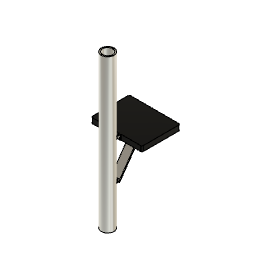
Seat_rod v5 (Autodesk Fusion 360 design; units mm, degrees)
Autodesk Fusion 360 part; units mm, degrees
sketch "草图1" plane through (0, 0, 0) normal (0, 0, 1) x (1, 0, 0)
  circle A0 centre (0, 0) radius 25
  dimension "d1" = 50
  constraint coincident A0.centre origin
  measures "d1" diameter of A0
extrude "拉伸1" add sketch "草图1" along normal mid plane 600 makes body 1
sketch "草图2" plane through (0, 0, 0) normal (0, 0, 1) x (1, 0, 0)
  line L0 (-10, 23) -> (-10, 35)
  line L1 (-10, 35) -> (10, 35)
  line L2 (10, 35) -> (10, 23)
  circle A0 centre (0, 0) radius 25
  circle A1 centre (0, 0) radius 25.0799
  dimension "d4" = 12
  dimension "d5" = 20
  dimension "d6" = 35
  dimension "d7" = 23
  dimension "d8" = 10
  constraint vertical L0
  constraint perpendicular L0 L1
  constraint perpendicular L1 L2
  constraint concentric A0 A1
  constraint coincident L2.end A1
  measures "d4" distance of L1.end L2.end
  measures "d5" distance of L0.end L1.end
  measures "d6" distance of A0.centre L1
  measures "d7" vertical distance of A0.centre L0.start
  measures "d8" horizontal distance of A0.centre L0.start
extrude "拉伸2" add sketch "草图2" along normal mid plane 12 separate body contours L0 L1 L2 A1 makes body 2
sketch "草图3" plane through (-10, 0, 0) normal (-1, 0, 0) x (0, -1, 0)
  line L0 (-23, -6) -> (-23, 6)
  line L1 (-23, 6) -> (-35, 6)
  line L2 (-35, 6) -> (-35, -6)
  line L3 (-35, -6) -> (-23, -6)
  circle A0 centre (-30, 0) radius 3
  line L4 (-1.75, 0) -> (-22.5, 0)
  dimension "d11" = 6
  dimension "d12" = 30
  constraint coincident A0.centre L4
  measures "d11" diameter of A0
  measures "d12" distance of origin A0.centre
extrude "拉伸3" cut sketch "草图3" against normal blind 20 contours A0 bodies 2
fillet "圆角1" radius 6 2 edges at (0, 35, 6) (0, 35, -6) on bodies 2
sketch "草图1 (2)" plane through (0, 0, 0) normal (1, 0, 0) x (0, 1, 0) in component "椅子"
  circle A0 centre (30, 0) radius 3
extrude "拉伸1'" add sketch "草图1 (2)" along normal mid plane 36 separate body makes body 3 in component "椅子"
sketch "草图1 (3)" plane through (0, 0, 0) normal (1, 0, 0) x (0, 1, 0) in component "支撑"
ref_plane "工作平面1" through (0, 0, -150) normal (0, 0, 1) x (1, 0, 0)
sketch "草图4" plane through (0, 0, -150) normal (0, 0, 1) x (1, 0, 0)
  circle A0 centre (0, 0) radius 25
  line L0 (-10, 29) -> (10, 29)
  line L1 (10, 29) -> (10, 23)
  arc A1 (10, 23) -> (-10, 23) centre (0, 0) ccw
  line L2 (-10, 23) -> (-10, 29)
  line L3 (-10, 29) -> (-10, 35)
  line L4 (-10, 29) -> (10, 29)
  line L5 (10, 35) -> (10, 29)
  line L6 (10, 29) -> (-10, 29)
  line L7 (10, 35) -> (-10, 35)
  constraint coincident L5.start L7.start
  constraint coincident L3.end L7.end
extrude "拉伸4" add sketch "草图4" along normal mid plane 10 separate body contours L0 L3 L4 L5 L6 L7 | L0 L1 A1 L2 L4 L6 makes body 4
sketch "草图8" plane through (0, 0, 0) normal (0, 0, 1) x (1, 0, 0) in component "椅子"
  line L0 (-10, 29) -> (-10, 35)
  line L1 (-10, 29) -> (10, 29)
  line L2 (10, 35) -> (10, 29)
  line L3 (10, 29) -> (-10, 29)
  line L4 (18, 33) -> (18, 35)
  line L5 (18, 35) -> (100, 35)
  line L6 (100, 35) -> (100, 185)
  line L7 (100, 185) -> (-100, 185)
  line L8 (-100, 185) -> (-100, 35)
  line L9 (-100, 35) -> (-18, 35)
  line L10 (-18, 35) -> (-18, 33)
  line L11 (-18, 33) -> (-10, 33)
  line L12 (-10, 35) -> (10, 35)
  line L13 (10, 33) -> (18, 33)
  line L14 (0, 1.75) -> (0, 22.5)
  dimension "d65" = 200
  dimension "d67" = 2
  dimension "d68" = 2
  dimension "d69" = 82
  dimension "d70" = 82
  dimension "d71" = 35
  dimension "d72" = 185
  dimension "d73" = 35
  constraint perpendicular L3 L4
  constraint perpendicular L4 L5
  constraint perpendicular L3 L6
  constraint perpendicular L8 L9
  constraint perpendicular L9 L10
  constraint coincident L0 L11.end
  constraint perpendicular L0 L11
  constraint coincident L0.end L12.start
  constraint coincident L2.start L12.end
  constraint coincident L2 L13.start
  constraint perpendicular L4 L13
  constraint symmetric L6 L8 L14
  constraint parallel L7 L9
  measures "d65" distance of L6.end L7.end
  measures "d67" distance of L9.end L10.end
  measures "d68" distance of L4.start L4.end
  measures "d69" distance of L4.end L5.end
  measures "d70" distance of L8.end L9.end
  measures "d71" distance of origin L9
  measures "d72" distance of origin L7
  measures "d73" distance of L5 origin
extrude "拉伸5" add sketch "草图8" along normal mid plane 20 separate body contours L0 L2 L4 L5 L6 L7 L8 L9 L10 L11 L12 L13 makes body 5 in component "椅子"
fillet "圆角4" radius 5 4 edges at (-100, 35, 0) (-100, 185, 0) (100, 185, 0) (100, 35, 0) on bodies 5 in component "椅子"
fillet "圆角2" radius 5 2 edges at (0, 35, -145) (0, 35, -155) on bodies 4
sketch "草图5" plane through (-10, 0, 0) normal (-1, 0, 0) x (0, -1, 0)
  arc A0 (-30, -145) -> (-30, -155) centre (-30, -150) ccw
  line L0 (-30, -155) -> (-23, -155)
  line L1 (-23, -155) -> (-23, -145)
  line L2 (-23, -145) -> (-30, -145)
  circle A1 centre (-30, -150) radius 2.5
  dimension "d80" = 5
  constraint concentric A0 A1
  measures "d80" diameter of A1
extrude "拉伸5'" cut sketch "草图5" against normal blind 20 contours A1 bodies 4
sketch "草图2 (2)" plane through (0, 0, 0) normal (1, 0, 0) x (0, 1, 0) in component "支撑"
  circle A0 centre (30, -150) radius 2.5
  arc A1 (30, -155) -> (30, -145) centre (30, -150) ccw
  line L0 (30, -155) -> (23, -155)
  line L1 (23, -155) -> (23, -145)
  line L2 (23, -145) -> (30, -145)
extrude "拉伸1''" add sketch "草图2 (2)" along normal mid plane 32 separate body contours A0 makes body 6 in component "支撑"
sketch "草图3 (2)" plane through (0, 0, 0) normal (1, 0, 0) x (0, 1, 0) in component "支撑"
  circle A0 centre (30, -150) radius 2.5
  line L0 (32.0551, -151.4236) -> (126.0146, -15.7895)
  line L1 (27.9449, -148.5764) -> (121.9045, -12.9423)
  circle A1 centre (123.9595, -14.3659) radius 2.5
  line L2 (30, -145) -> (23, -145)
  line L3 (123.9595, -11.8659) -> (153.9595, -11.8659)
  line L4 (123.9595, -16.8659) -> (153.9595, -16.8659)
  circle A2 centre (153.9595, -14.3659) radius 2.5
  line L5 (31.9311, -142.8222) -> (36.0412, -145.6695)
  dimension "d85" = 165
  dimension "d86" = 165
  dimension "d87" = 124.712
  dimension "d88" = 30
  dimension "d89" = 30
  dimension "d90" = 7
  constraint coincident A0 L0.start
  constraint coincident A0 L1.start
  constraint parallel L0 L1
  constraint tangent A0 L1
  constraint tangent A0 L0
  constraint coincident L1.end A1
  constraint tangent L1 A1
  constraint coincident L0.end A1
  constraint coincident A1 L3.start
  constraint horizontal L3
  constraint coincident A1 L4.start
  constraint horizontal L4
  constraint tangent A1 L3
  constraint tangent A1 L4
  constraint coincident L4.end A2
  constraint tangent L4 A2
  constraint coincident L3.end A2
  constraint coincident L1 L5.start
  constraint coincident L0 L5.end
  constraint perpendicular L0 L5
  measures "d85" distance of L1.start L1.end
  measures "d86" distance of L0.start L0.end
  measures "d87" angle of L1 L2
  measures "d88" distance of L3.start L3.end
  measures "d89" distance of L4.start L4.end
  measures "d90" distance of A0.centre L5
extrude "拉伸2'" add sketch "草图3 (2)" along normal mid plane 32 separate body contours L0 L1 A1 L4 L5 | A1 | L0 A1 L4 | L0 A1 L3 L4 A2 | A2 makes body 7 in component "支撑"
sketch "草图4 (2)" plane through (0, -56.5011, -81.5614) normal (0, -0.569452, -0.822025) x (1, 0, 0) in component "支撑"
  line L0 (-16, -112.5785) -> (16, -112.5785)
  line L1 (16, -112.5785) -> (16, -107.5785)
  line L2 (16, -107.5785) -> (-16, -107.5785)
  line L3 (-16, -107.5785) -> (-16, -112.5785)
  line L4 (10, -107.5785) -> (10, -112.5785)
  line L5 (10, -107.2312) -> (10, -115.0785)
  line L6 (10, -107.2312) -> (10, -101.4771)
  line L7 (10, -101.4771) -> (10, -107.1716)
  line L8 (10, -107.1716) -> (10, -112.9258)
  line L9 (10, -112.5785) -> (16, -112.5785)
  line L10 (16, -107.5785) -> (10, -107.5785)
  line L11 (-16, -112.5785) -> (-10, -112.5785)
  line L12 (-10, -112.5785) -> (-10, -107.5785)
  line L13 (-10, -107.5785) -> (-16, -107.5785)
  line L14 (-16, -107.5785) -> (-16, -112.5785)
  dimension "d93" = 20
  dimension "d94" = 5
  constraint coincident L4.end L9.start
  constraint coincident L0.end L1.start
  constraint coincident L1.end L2.start
  constraint coincident L4.start L10.end
  constraint horizontal L11
  constraint vertical L12
  constraint horizontal L13
  constraint vertical L14
  constraint coincident L0.start L3.end
  measures "d93" distance of L8 L12
  measures "d94" distance of L11 L13
extrude "拉伸3'" add sketch "草图4 (2)" along normal blind 7 contours L0 L2 L3 L11 L12 L13 L14 | L0 L1 L2 L4 L5 L8 L9 L10 bodies 6 7 in component "支撑"
sketch "草图9" plane through (0, 0, 0) normal (1, 0, 0) x (0, 1, 0) in component "椅子"
  arc A0 (123.9595, -11.8659) -> (121.9045, -12.9423) centre (123.9595, -14.3659) ccw
  line L0 (123.9595, -11.8659) -> (153.9595, -11.8659)
  arc A1 (153.9595, -16.8659) -> (153.9595, -11.8659) centre (153.9595, -14.3659) ccw
  line L1 (153.9595, -16.8659) -> (125.2689, -16.8659)
  line L2 (125.2689, -16.8659) -> (32.0551, -151.4236)
  arc A2 (27.9449, -148.5764) -> (32.0551, -151.4236) centre (30, -150) ccw
  line L3 (27.9449, -148.5764) -> (31.9311, -142.8222)
  line L4 (31.9311, -142.8222) -> (121.9045, -12.9423)
  line L5 (158, -10) -> (158, -17)
  line L6 (158, -17) -> (143, -17)
  line L7 (143, -17) -> (143, -22)
  line L8 (143, -22) -> (163, -22)
  line L9 (163, -22) -> (163, -10)
  line L10 (163, -10) -> (158, -10)
  dimension "d97" = 20
  dimension "d98" = 5
  dimension "d99" = 5
  dimension "d100" = 12
  dimension "d101" = 143
  dimension "d102" = 22
  constraint vertical L5
  constraint perpendicular L5 L6
  constraint perpendicular L6 L7
  constraint perpendicular L7 L8
  constraint perpendicular L8 L9
  constraint perpendicular L9 L10
  measures "d97" distance of L7.end L8.end
  measures "d98" distance of L6.end L7.end
  measures "d99" distance of L5 L9
  measures "d100" distance of L8.end L9.end
  measures "d101" distance of origin L7
  measures "d102" distance of origin L8
extrude "拉伸6" add sketch "草图9" along normal mid plane 32 separate body contours L5 L6 L7 L8 L9 L10 makes body 8 in component "椅子"
fillet "圆角5" radius 2.5 2 edges at (0, 163, -22) (0, 143, -22) on bodies 8 in component "椅子"
sketch "草图6" plane through (0, 0, 300) normal (0, 0, 1) x (-1, 0, 0)
  circle A0 centre (0, 0) radius 25
  circle A1 centre (0, 0) radius 20
  dimension "d107" = 40
  constraint concentric A0 A1
  measures "d107" diameter of A1
extrude "拉伸6'" cut sketch "草图6" against normal through all contours A1 bodies 1
component "椅子" placed x (1, 0, 0) y (0, 1, 0) z (0, 0, 1) at (0, 0, 0)
component "支撑" placed x (1, 0, 0) y (0, 1, 0) z (0, 0, 1) at (0, 0, 0)
